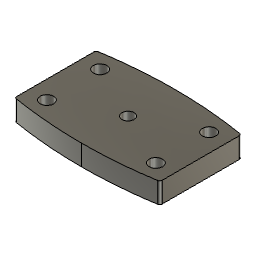
Minx adapterit v5 (Autodesk Fusion 360 design; units mm, degrees)
Autodesk Fusion 360 part; units mm, degrees
sketch "basePlate" plane through (0, 0, 0) normal (0, 0, 1) x (1, 0, 0)
  line L0 (-31.1665, 19.7211) -> (28.8335, 19.7211)
  line L1 (28.8335, 19.7211) -> (28.8335, -18.7789)
  line L2 (28.8335, -18.7789) -> (-31.1665, -18.7789)
  line L3 (-31.1665, -18.7789) -> (-31.1665, 19.7211)
  circle A0 centre (-23.6665, 11.4711) radius 2.75
  line L4 (-1.1665, 19.7211) -> (-1.1665, -18.7789)
  line L5 (28.8335, 19.7211) -> (28.8335, 17.2211)
  arc A1 (28.8335, 17.2211) -> (-1.1665, 19.7211) centre (-1.1742, -161.6214) ccw
  arc A2 (-1.1665, 19.7211) -> (-31.1665, 17.2211) centre (-1.1588, -161.6214) ccw
  line L6 (-31.1665, 0.4711) -> (28.8335, 0.4711)
  arc A3 (-31.1665, -16.2789) -> (-1.1665, -18.7789) centre (-1.1588, 162.5637) ccw
  arc A4 (-1.1665, -18.7789) -> (28.8335, -16.2789) centre (-1.1742, 162.5637) ccw
  circle A5 centre (-23.6665, -10.5289) radius 2.75
  circle A6 centre (21.3335, 11.4711) radius 2.75
  circle A7 centre (21.3335, -10.5289) radius 2.75
  dimension "d1" = 60
  dimension "d2" = 38.5
  dimension "d3" = 5.5
  dimension "d6" = 2.5
  dimension "d7" = 7.5
  dimension "d10" = 22
  constraint horizontal L0
  constraint vertical L1
  constraint horizontal L2
  constraint vertical L3
  constraint midpoint L0 L4.start
  constraint midpoint L2 L4.end
  constraint perpendicular L0 L5
  constraint tangent L0 A1
  constraint symmetric A1.end L4 A2.start
  constraint symmetric L4 L5.end A2.end
  constraint symmetric L4 A1 A2
  constraint midpoint L3 L6.start
  constraint midpoint L1 L6.end
  constraint symmetric L4.start L6 L4.end
  constraint symmetric L5.end L6 A4.end
  constraint symmetric A1 L6 A4
  constraint symmetric A2.end L6 A3.start
  constraint symmetric A2 L6 A3
  constraint symmetric A0 L6 A5
  constraint symmetric A0 L4 A6
  constraint symmetric L4 A5 A7
  measures "d1" distance of L0.start L0.end
  measures "d2" distance of L0.start L2.end
  measures "d3" diameter of A0
  measures "d6" distance of L0.end L5.end
  measures "d7" distance of L3 A0.centre
extrude "Extrude1" add sketch "basePlate" along normal blind 8.5 contours L1 L4 A1 L6 | L3 L4 A2 L6 | L1 L4 L6 A4 | L3 L4 L6 A3 makes body 1
fillet "Fillet1" radius 1 1 edges at (28.8335, -16.2789, 4.25) on bodies 1
fillet "Fillet2" radius 1 1 edges at (28.8335, 17.2211, 4.25) on bodies 1
fillet "Fillet3" radius 1 1 edges at (-31.1665, 17.2211, 4.25) on bodies 1
fillet "Fillet4" radius 1 1 edges at (-31.1665, -16.2789, 4.25) on bodies 1
sketch "groove" plane through (28.8335, 0, 0) normal (1, 0, 0) x (0, 1, 0)
  line L0 (16.3729, 0) -> (16.3729, 8.5)
  line L1 (16.3729, 8.5) -> (-15.4307, 8.5)
  line L2 (-15.4307, 8.5) -> (-15.4307, 0)
  line L3 (-15.4307, 0) -> (16.3729, 0)
  line L4 (0.4711, 8.5) -> (0.4711, 0)
  line L5 (0.4711, 8.5) -> (0.4711, 13.5)
  line L6 (0.4711, 8.5) -> (5.4711, 8.5)
  line L7 (0.4711, 13.5) -> (5.4711, 8.5)
  line L8 (0.4711, 8.5) -> (-4.5289, 8.5)
  line L9 (0.4711, 13.5) -> (-4.5289, 8.5)
  dimension "d26" = 5
  dimension "d27" = 5
  constraint midpoint L1 L4.start
  constraint midpoint L3 L4.end
  constraint perpendicular L1 L5
  constraint perpendicular L4 L6
  constraint symmetric L4.start L5 L6.start
  constraint symmetric L7.start L5 L9.start
  constraint symmetric L5 L6.end L8.end
  measures "d26" distance of L4.start L5.end
  measures "d27" distance of L4.start L6.end
extrude "Extrude2" add sketch "groove" against normal blind 60 separate body contours L1 L5 L6 L7 | L1 L5 L8 L9 makes body 2
fillet "Fillet5" radius 1 1 edges at (-1.1665, 0.4711, 13.5) on bodies 2
hole "Hole1" at (-1.1665, 0.4711, 0) direction (0, 0, 1) diameter 5 depth 13.5 tip angle 180 counterbore diameter 8.5 counterbore depth 4.25 bodies 1 2
combine "Combine1" operation add target body 1 tool bodies 2 keep tools result as body 3 in component "mountAssembly"
component "mountAssembly" placed x (1, 0, 0) y (0, 1, 0) z (0, 0, 1) at (0, 0, 0)
hidden bodies 2
equation "d1 = basePlateWidth"
equation "d2 = basePlateHeighth"
equation "d3 = screwHoleDiameter"
equation "d7 = screwHoleCenterFromBorder"
equation "screwHoleDiameter = 5.5 mm" comment "Hole diameter for heat insert"
equation "d11 = basePlateExtrude"
equation "cornerRoundRad = 1 mm" comment "Smoothing of base plate corners"
equation "d15 = cornerRoundRad"
equation "d17 = cornerRoundRad"
equation "d19 = cornerRoundRad"
equation "d21 = cornerRoundRad"
equation "basePlateExtrude = 8.5 mm" comment "Square base plate extrude (heat insert) height"
equation "screwHoleCenterFromBorder = 7.5 mm" comment "How far heat insert hole center is from base plate border"
equation "basePlateHeighth = 38.5 mm"
equation "basePlateWidth = 60 mm"
equation "d26 = grooveDepth"
equation "d27 = grooveWidth / 2"
equation "grooveDepth = 5 mm"
equation "grooveWidth = 10 mm"
equation "d30 = -basePlateWidth"
equation "d33 = cornerRoundRad"
equation "d34 = basePlateExtrude + grooveDepth"
equation "d35 = wallScrewDiameter"
equation "d37 = basePlateExtrude / 2"
equation "d38 = wallScrewBase"
equation "wallScrewDiameter = 5 mm"
equation "wallScrewBase = 8.5 mm"
named bodies: "basePlate", "groove", "mountAssembly"
